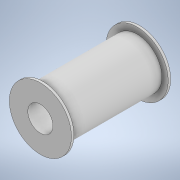
# Autodesk Inventor part: Seil_Rolle_Antrieb
Saved by Autodesk Inventor 2021 (Build 250183000, 183)
## iProperties
Created: 2022-06-29
Part Number: Seil_Rolle_Antrieb
Material: Generisch
Document SubType Name: Modeling
Designer: adria
Mass: 9.71506 g
Surface Area: 49.8883 cm^2
Volume: 9.71506 cm^3
Density: 1 g/cm^3
Appearance: Vorgabe
Author: adria
Autodesk Inventor part; units mm, degrees
ref_plane "YZ Plane" through (0, 0, 0) normal (1, 0, 0) x (0, 1, 0)
ref_plane "XZ Plane" through (0, 0, 0) normal (0, 1, 0) x (-1, 0, 0)
ref_plane "XY Plane" through (0, 0, 0) normal (0, 0, 1) x (1, 0, 0)
sketch "Skizze1" plane through (0, 0, 0) normal (0, 1, 0) x (-1, 0, 0)
  line L0 (0, 20) -> (12.5, 20)
  line L1 (12.5, 20) -> (12.5, 19)
  line L2 (12.5, 19) -> (10, 19)
  line L3 (10, 19) -> (10, -19)
  line L4 (10, -19) -> (12.5, -19)
  line L5 (12.5, -19) -> (12.5, -20)
  line L6 (12.5, -20) -> (0, -20)
  line L7 (0, 20) -> (0, -20)
  line L8 (15, 0) -> (-2.5, 0) projected
  line L9 (0, -28) -> (0, 28) projected
  point P0 (0, 0)
  dimension "d4" = 20
  dimension "d5" = 25
  dimension "d6" = 40
  dimension "d7" = 1
  constraints: 16 end point, 4 horizontal, 2 point on line, 2 vertical, 1 midpoint, 1 perpendicular, 2 other
  measures "d4" diameter of L3 L9
  measures "d5" diameter of L5 L9
  measures "d6" distance of L0.start L6.end
  measures "d7" distance of L4.end L5.end
revolve "Umdrehung1" add sketch "Skizze1" angle 360 about axis through (0, 0, 20) along (0, 0, -1)
sketch "Skizze2" plane through (0, 0, 20) normal (0, 0, 1) x (1, 0, 0)
  circle A0 centre (0, 0) radius 12.5 projected
  circle A1 centre (0, 0) radius 5.05
  dimension "d1" = 10.1
  constraints: 1 centre point, 1 coincident
  measures "d1" diameter of A1
extrude "Extrusion1" cut sketch "Skizze2" against normal through all contours A1
